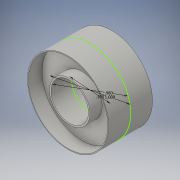
# Autodesk Inventor part: plastic idler wheel base part
Saved by Autodesk Inventor 2016 (Build 200138000, 138)
## iProperties
Created: 2015-10-09
Part Number: plastic idler wheel base part
Material: Generic
Document SubType Name: Modeling
Designer: Delta
Density: 1 g/cm^3
Appearance: Default
Author: Delta
Autodesk Inventor part; units mm, degrees
ref_plane "YZ Plane" through (0, 0, 0) normal (1, 0, 0) x (0, 1, 0)
ref_plane "XZ Plane" through (0, 0, 0) normal (0, 1, 0) x (-1, 0, 0)
ref_plane "XY Plane" through (0, 0, 0) normal (0, 0, 1) x (1, 0, 0)
sketch "Sketch1" plane through (0, 0, 0) normal (0, 0, 1) x (1, 0, 0)
  circle A0 centre (0, 0) radius 12.7
  circle A1 centre (0, 0) radius 12.446
  circle A2 centre (0, 0) radius 6.35
  circle A3 centre (0, 0) radius 5.8601
  dimension "d1" = 25.4
  dimension "d2" = 24.892
  dimension "d3" = 12.7
  constraints: 4 centre point, 3 coincident
  measures "d1" diameter of A0
  measures "d2" diameter of A1
  measures "d3" diameter of A2
extrude "Extrusion1" [suppressed]
extrude "Extrusion2" add sketch "Sketch1" along normal blind 6.858 and the other way blind 6.858 contours A0
extrude "Extrusion3" add sketch "Sketch1" along normal blind 2.54 and the other way blind 2.54 contours A1
extrude "Extrusion4" add sketch "Sketch1" along normal blind 6.35 and the other way blind 6.35 contours A2
fillet "Fillet1" [suppressed]
body "Solid1"
